Autodesk Fusion 360 part; units mm, degrees
(part 2 of 2)
sketch "Sketch13" plane through (0, 16, 0) normal (0, 1, 0) x (-1, 0, 0)
  arc A0 (-64.7977, -91.0875) -> (-65.2878, -90.2878) centre (-68, -92.5) ccw
  line L0 (-64.7977, -91.0875) -> (-65.3533, -91.0875)
  arc A1 (-65.3533, -91.0875) -> (-65.6435, -90.6435) centre (-68, -92.5) ccw
  line L1 (-65.6435, -90.6435) -> (-65.2878, -90.2878)
  arc A2 (-63.869, -96.131) -> (-62.7085, -94) centre (-68, -92.5) ccw
  line L2 (-63.869, -96.131) -> (-64.2233, -95.7767)
  arc A3 (-64.2233, -95.7767) -> (-63.2303, -94) centre (-68, -92.5) ccw
  line L3 (-63.2303, -94) -> (-62.7085, -94)
  arc A4 (-71.631, -96.631) -> (-64.369, -96.631) centre (-68, -92.5) ccw
  line L4 (-71.631, -96.631) -> (-71.2767, -96.2767)
  arc A5 (-71.2767, -96.2767) -> (-64.7233, -96.2767) centre (-68, -92.5) ccw
  line L5 (-64.7233, -96.2767) -> (-64.369, -96.631)
  line L6 (-69.9125, -91.0875) -> (-70.0627, -91.0875)
  arc A6 (-70, -91) -> (-70.0627, -91.0875) centre (-68, -92.5) ccw
  line L7 (-70, -91) -> (-69.9125, -91.0875)
  line L8 (-67.4952, -91.0875) -> (-68.5048, -91.0875)
  arc A7 (-67.4952, -91.0875) -> (-68.5048, -91.0875) centre (-68, -92.5) ccw
  arc A8 (-64.369, -88.369) -> (-71.631, -88.369) centre (-68, -92.5) ccw
  line L9 (-64.369, -88.369) -> (-64.7233, -88.7233)
  arc A9 (-64.7233, -88.7233) -> (-71.2767, -88.7233) centre (-68, -92.5) ccw
  line L10 (-71.2767, -88.7233) -> (-71.631, -88.369)
  arc A10 (-58.9221, -95.9221) -> (-53.0779, -95.9221) centre (-56, -92.5) ccw
  line L11 (-58.9221, -95.9221) -> (-58.5674, -95.5674)
  arc A11 (-58.5674, -95.5674) -> (-53.4326, -95.5674) centre (-56, -92.5) ccw
  line L12 (-53.4326, -95.5674) -> (-53.0779, -95.9221)
  arc A12 (-60.2426, -94) -> (-59.4221, -95.4221) centre (-56, -92.5) ccw
  line L13 (-60.2426, -94) -> (-59.7081, -94)
  arc A13 (-59.7081, -94) -> (-59.0674, -95.0674) centre (-56, -92.5) ccw
  line L14 (-59.0674, -95.0674) -> (-59.4221, -95.4221)
  line L15 (-43.4952, -91.0875) -> (-44.5048, -91.0875)
  arc A14 (-43.4952, -91.0875) -> (-44.5048, -91.0875) centre (-44, -92.5) ccw
  line L16 (-54.0875, -91.0875) -> (-54, -91)
  arc A15 (-53.9373, -91.0875) -> (-54, -91) centre (-56, -92.5) ccw
  line L17 (-53.9373, -91.0875) -> (-54.0875, -91.0875)
  arc A16 (-51.869, -96.131) -> (-50.7085, -94) centre (-56, -92.5) ccw
  line L18 (-51.869, -96.131) -> (-52.2233, -95.7767)
  arc A17 (-52.2233, -95.7767) -> (-51.2303, -94) centre (-56, -92.5) ccw
  line L19 (-51.2303, -94) -> (-50.7085, -94)
  arc A18 (-52.369, -88.369) -> (-59.631, -88.369) centre (-56, -92.5) ccw
  line L20 (-52.369, -88.369) -> (-52.7233, -88.7233)
  arc A19 (-52.7233, -88.7233) -> (-59.2767, -88.7233) centre (-56, -92.5) ccw
  line L21 (-59.2767, -88.7233) -> (-59.631, -88.369)
  line L22 (-41.9373, -91.0875) -> (-42.0875, -91.0875)
  line L23 (-42.0875, -91.0875) -> (-42, -91)
  arc A20 (-41.9373, -91.0875) -> (-42, -91) centre (-44, -92.5) ccw
  line L24 (-45.9125, -91.0875) -> (-46.0627, -91.0875)
  arc A21 (-46, -91) -> (-46.0627, -91.0875) centre (-44, -92.5) ccw
  line L25 (-46, -91) -> (-45.9125, -91.0875)
  arc A22 (-49.2915, -94) -> (-48.131, -96.131) centre (-44, -92.5) ccw
  line L26 (-49.2915, -94) -> (-48.7697, -94)
  arc A23 (-48.7697, -94) -> (-47.7767, -95.7767) centre (-44, -92.5) ccw
  line L27 (-47.7767, -95.7767) -> (-48.131, -96.131)
  arc A24 (-45.5, -94.5) -> (-42.5, -94.5) centre (-44, -92.5) ccw
  line L28 (-45.5, -94.5) -> (-45.1419, -94.1419)
  arc A25 (-45.1419, -94.1419) -> (-42.8581, -94.1419) centre (-44, -92.5) ccw
  line L29 (-42.8581, -94.1419) -> (-42.5, -94.5)
  arc A26 (-40.369, -88.369) -> (-47.631, -88.369) centre (-44, -92.5) ccw
  line L30 (-40.369, -88.369) -> (-40.7233, -88.7233)
  arc A27 (-40.7233, -88.7233) -> (-47.2767, -88.7233) centre (-44, -92.5) ccw
  line L31 (-47.2767, -88.7233) -> (-47.631, -88.369)
  arc A28 (-38.6845, -91.0875) -> (-39.869, -88.869) centre (-44, -92.5) ccw
  line L32 (-38.6845, -91.0875) -> (-39.2037, -91.0875)
  arc A29 (-39.2037, -91.0875) -> (-40.2233, -89.2233) centre (-44, -92.5) ccw
  line L33 (-40.2233, -89.2233) -> (-39.869, -88.869)
  arc A30 (-42.5, -90.5) -> (-45.5, -90.5) centre (-44, -92.5) ccw
  line L34 (-42.5, -90.5) -> (-42.8581, -90.8581)
  arc A31 (-42.8581, -90.8581) -> (-45.1419, -90.8581) centre (-44, -92.5) ccw
  line L35 (-45.1419, -90.8581) -> (-45.5, -90.5)
  arc A32 (-47.631, -96.631) -> (-40.369, -96.631) centre (-44, -92.5) ccw
  line L36 (-47.631, -96.631) -> (-47.2767, -96.2767)
  arc A33 (-47.2767, -96.2767) -> (-40.7233, -96.2767) centre (-44, -92.5) ccw
  line L37 (-40.7233, -96.2767) -> (-40.369, -96.631)
  arc A34 (-46.7122, -90.2878) -> (-47.2023, -91.0875) centre (-44, -92.5) ccw
  line L38 (-46.7122, -90.2878) -> (-46.3565, -90.6435)
  arc A35 (-46.3565, -90.6435) -> (-46.6467, -91.0875) centre (-44, -92.5) ccw
  line L39 (-46.6467, -91.0875) -> (-47.2023, -91.0875)
  arc A36 (-40.7977, -91.0875) -> (-41.2878, -90.2878) centre (-44, -92.5) ccw
  line L40 (-40.7977, -91.0875) -> (-41.3533, -91.0875)
  arc A37 (-41.3533, -91.0875) -> (-41.6435, -90.6435) centre (-44, -92.5) ccw
  line L41 (-41.6435, -90.6435) -> (-41.2878, -90.2878)
  arc A38 (-41.2878, -94.7122) -> (-40.8377, -94) centre (-44, -92.5) ccw
  line L42 (-41.2878, -94.7122) -> (-41.6435, -94.3565)
  arc A39 (-41.6435, -94.3565) -> (-41.4019, -94) centre (-44, -92.5) ccw
  line L43 (-41.4019, -94) -> (-40.8377, -94)
  arc A40 (-59.631, -96.631) -> (-52.369, -96.631) centre (-56, -92.5) ccw
  line L44 (-59.631, -96.631) -> (-59.2767, -96.2767)
  arc A41 (-59.2767, -96.2767) -> (-52.7233, -96.2767) centre (-56, -92.5) ccw
  line L45 (-52.7233, -96.2767) -> (-52.369, -96.631)
  arc A42 (-52.7977, -91.0875) -> (-53.2878, -90.2878) centre (-56, -92.5) ccw
  line L46 (-52.7977, -91.0875) -> (-53.3533, -91.0875)
  arc A43 (-53.3533, -91.0875) -> (-53.6435, -90.6435) centre (-56, -92.5) ccw
  line L47 (-53.6435, -90.6435) -> (-53.2878, -90.2878)
  arc A44 (-54.8581, -90.8581) -> (-57.1419, -90.8581) centre (-56, -92.5) ccw
  line L48 (-57.1419, -90.8581) -> (-57.5, -90.5)
  arc A45 (-54.5, -90.5) -> (-57.5, -90.5) centre (-56, -92.5) ccw
  line L49 (-54.5, -90.5) -> (-54.8581, -90.8581)
  line L50 (-57.9125, -91.0875) -> (-58.0627, -91.0875)
  arc A46 (-58, -91) -> (-58.0627, -91.0875) centre (-56, -92.5) ccw
  line L51 (-58, -91) -> (-57.9125, -91.0875)
  arc A47 (-58.2122, -95.2122) -> (-53.7878, -95.2122) centre (-56, -92.5) ccw
  line L52 (-58.2122, -95.2122) -> (-57.8565, -94.8565)
  arc A48 (-57.8565, -94.8565) -> (-54.1435, -94.8565) centre (-56, -92.5) ccw
  line L53 (-54.1435, -94.8565) -> (-53.7878, -95.2122)
  line L54 (-55.4952, -91.0875) -> (-56.5048, -91.0875)
  arc A49 (-55.4952, -91.0875) -> (-56.5048, -91.0875) centre (-56, -92.5) ccw
  arc A50 (-66.8581, -90.8581) -> (-69.1419, -90.8581) centre (-68, -92.5) ccw
  line L55 (-69.1419, -90.8581) -> (-69.5, -90.5)
  arc A51 (-66.5, -90.5) -> (-69.5, -90.5) centre (-68, -92.5) ccw
  line L56 (-66.5, -90.5) -> (-66.8581, -90.8581)
  arc A52 (-70.7122, -90.2878) -> (-71.2023, -91.0875) centre (-68, -92.5) ccw
  line L57 (-70.7122, -90.2878) -> (-70.3565, -90.6435)
  arc A53 (-70.3565, -90.6435) -> (-70.6467, -91.0875) centre (-68, -92.5) ccw
  line L58 (-70.6467, -91.0875) -> (-71.2023, -91.0875)
  arc A54 (-71.1623, -94) -> (-70.7122, -94.7122) centre (-68, -92.5) ccw
  line L59 (-71.1623, -94) -> (-70.5981, -94)
  arc A55 (-70.5981, -94) -> (-70.3565, -94.3565) centre (-68, -92.5) ccw
  line L60 (-70.3565, -94.3565) -> (-70.7122, -94.7122)
  arc A56 (-69.5, -94.5) -> (-66.5, -94.5) centre (-68, -92.5) ccw
  line L61 (-69.5, -94.5) -> (-69.1419, -94.1419)
  arc A57 (-69.1419, -94.1419) -> (-66.8581, -94.1419) centre (-68, -92.5) ccw
  line L62 (-66.8581, -94.1419) -> (-66.5, -94.5)
  line L63 (-66.0875, -91.0875) -> (-66, -91)
  arc A58 (-65.9373, -91.0875) -> (-66, -91) centre (-68, -92.5) ccw
  line L64 (-65.9373, -91.0875) -> (-66.0875, -91.0875)
  arc A59 (-63.7274, -91.0875) -> (-64.5779, -89.5779) centre (-68, -92.5) ccw
  line L65 (-63.7274, -91.0875) -> (-64.2577, -91.0875)
  arc A60 (-64.2577, -91.0875) -> (-64.9326, -89.9326) centre (-68, -92.5) ccw
  line L66 (-64.9326, -89.9326) -> (-64.5779, -89.5779)
  arc A61 (-64.5779, -95.4221) -> (-63.7574, -94) centre (-68, -92.5) ccw
  line L67 (-64.5779, -95.4221) -> (-64.9326, -95.0674)
  arc A62 (-64.9326, -95.0674) -> (-64.2919, -94) centre (-68, -92.5) ccw
  line L68 (-64.2919, -94) -> (-63.7574, -94)
  arc A63 (-70.9221, -95.9221) -> (-65.0779, -95.9221) centre (-68, -92.5) ccw
  line L69 (-70.9221, -95.9221) -> (-70.5674, -95.5674)
  arc A64 (-70.5674, -95.5674) -> (-65.4326, -95.5674) centre (-68, -92.5) ccw
  line L70 (-65.4326, -95.5674) -> (-65.0779, -95.9221)
  arc A65 (-73.2915, -94) -> (-72.131, -96.131) centre (-68, -92.5) ccw
  line L71 (-73.2915, -94) -> (-72.7697, -94)
  arc A66 (-72.7697, -94) -> (-71.7767, -95.7767) centre (-68, -92.5) ccw
  line L72 (-71.7767, -95.7767) -> (-72.131, -96.131)
  arc A67 (-72.131, -88.869) -> (-73.3155, -91.0875) centre (-68, -92.5) ccw
  line L73 (-72.131, -88.869) -> (-71.7767, -89.2233)
  arc A68 (-71.7767, -89.2233) -> (-72.7963, -91.0875) centre (-68, -92.5) ccw
  line L74 (-72.7963, -91.0875) -> (-73.3155, -91.0875)
  arc A69 (-65.4326, -89.4326) -> (-70.5674, -89.4326) centre (-68, -92.5) ccw
  line L75 (-70.5674, -89.4326) -> (-70.9221, -89.0779)
  arc A70 (-65.0779, -89.0779) -> (-70.9221, -89.0779) centre (-68, -92.5) ccw
  line L76 (-65.0779, -89.0779) -> (-65.4326, -89.4326)
  arc A71 (-52.5779, -95.4221) -> (-51.7574, -94) centre (-56, -92.5) ccw
  line L77 (-52.5779, -95.4221) -> (-52.9326, -95.0674)
  arc A72 (-52.9326, -95.0674) -> (-52.2919, -94) centre (-56, -92.5) ccw
  line L78 (-52.2919, -94) -> (-51.7574, -94)
  arc A73 (-59.1623, -94) -> (-58.7122, -94.7122) centre (-56, -92.5) ccw
  line L79 (-59.1623, -94) -> (-58.5981, -94)
  arc A74 (-58.5981, -94) -> (-58.3565, -94.3565) centre (-56, -92.5) ccw
  line L80 (-58.3565, -94.3565) -> (-58.7122, -94.7122)
  arc A75 (-59.4221, -89.5779) -> (-60.2726, -91.0875) centre (-56, -92.5) ccw
  line L81 (-59.4221, -89.5779) -> (-59.0674, -89.9326)
  arc A76 (-59.0674, -89.9326) -> (-59.7423, -91.0875) centre (-56, -92.5) ccw
  line L82 (-59.7423, -91.0875) -> (-60.2726, -91.0875)
  arc A77 (-53.4326, -89.4326) -> (-58.5674, -89.4326) centre (-56, -92.5) ccw
  line L83 (-58.5674, -89.4326) -> (-58.9221, -89.0779)
  arc A78 (-53.0779, -89.0779) -> (-58.9221, -89.0779) centre (-56, -92.5) ccw
  line L84 (-53.0779, -89.0779) -> (-53.4326, -89.4326)
  arc A79 (-50.6845, -91.0875) -> (-51.869, -88.869) centre (-56, -92.5) ccw
  line L85 (-50.6845, -91.0875) -> (-51.2037, -91.0875)
  arc A80 (-51.2037, -91.0875) -> (-52.2233, -89.2233) centre (-56, -92.5) ccw
  line L86 (-52.2233, -89.2233) -> (-51.869, -88.869)
  arc A81 (-60.131, -88.869) -> (-61.3155, -91.0875) centre (-56, -92.5) ccw
  line L87 (-60.131, -88.869) -> (-59.7767, -89.2233)
  arc A82 (-59.7767, -89.2233) -> (-60.7963, -91.0875) centre (-56, -92.5) ccw
  line L88 (-60.7963, -91.0875) -> (-61.3155, -91.0875)
  arc A83 (-39.7274, -91.0875) -> (-40.5779, -89.5779) centre (-44, -92.5) ccw
  line L89 (-39.7274, -91.0875) -> (-40.2577, -91.0875)
  arc A84 (-40.2577, -91.0875) -> (-40.9326, -89.9326) centre (-44, -92.5) ccw
  line L90 (-40.9326, -89.9326) -> (-40.5779, -89.5779)
  arc A85 (-47.1623, -94) -> (-46.7122, -94.7122) centre (-44, -92.5) ccw
  line L91 (-47.1623, -94) -> (-46.5981, -94)
  arc A86 (-46.5981, -94) -> (-46.3565, -94.3565) centre (-44, -92.5) ccw
  line L92 (-46.3565, -94.3565) -> (-46.7122, -94.7122)
  arc A87 (-48.131, -88.869) -> (-49.3155, -91.0875) centre (-44, -92.5) ccw
  line L93 (-48.131, -88.869) -> (-47.7767, -89.2233)
  arc A88 (-47.7767, -89.2233) -> (-48.7963, -91.0875) centre (-44, -92.5) ccw
  line L94 (-48.7963, -91.0875) -> (-49.3155, -91.0875)
  arc A89 (-46.2122, -95.2122) -> (-41.7878, -95.2122) centre (-44, -92.5) ccw
  line L95 (-46.2122, -95.2122) -> (-45.8565, -94.8565)
  arc A90 (-45.8565, -94.8565) -> (-42.1435, -94.8565) centre (-44, -92.5) ccw
  line L96 (-42.1435, -94.8565) -> (-41.7878, -95.2122)
  arc A91 (-41.0779, -89.0779) -> (-46.9221, -89.0779) centre (-44, -92.5) ccw
  line L97 (-41.0779, -89.0779) -> (-41.4326, -89.4326)
  arc A92 (-41.4326, -89.4326) -> (-46.5674, -89.4326) centre (-44, -92.5) ccw
  line L98 (-46.5674, -89.4326) -> (-46.9221, -89.0779)
  arc A93 (-39.869, -96.131) -> (-38.7085, -94) centre (-44, -92.5) ccw
  line L99 (-39.869, -96.131) -> (-40.2233, -95.7767)
  arc A94 (-40.2233, -95.7767) -> (-39.2303, -94) centre (-44, -92.5) ccw
  line L100 (-39.2303, -94) -> (-38.7085, -94)
  arc A95 (-41.7878, -89.7878) -> (-46.2122, -89.7878) centre (-44, -92.5) ccw
  line L101 (-41.7878, -89.7878) -> (-42.1435, -90.1435)
  arc A96 (-42.1435, -90.1435) -> (-45.8565, -90.1435) centre (-44, -92.5) ccw
  line L102 (-45.8565, -90.1435) -> (-46.2122, -89.7878)
  arc A97 (-46.9221, -95.9221) -> (-41.0779, -95.9221) centre (-44, -92.5) ccw
  line L103 (-46.9221, -95.9221) -> (-46.5674, -95.5674)
  arc A98 (-46.5674, -95.5674) -> (-41.4326, -95.5674) centre (-44, -92.5) ccw
  line L104 (-41.4326, -95.5674) -> (-41.0779, -95.9221)
  arc A99 (-47.4221, -89.5779) -> (-48.2726, -91.0875) centre (-44, -92.5) ccw
  line L105 (-47.4221, -89.5779) -> (-47.0674, -89.9326)
  arc A100 (-47.0674, -89.9326) -> (-47.7423, -91.0875) centre (-44, -92.5) ccw
  line L106 (-47.7423, -91.0875) -> (-48.2726, -91.0875)
  arc A101 (-48.2426, -94) -> (-47.4221, -95.4221) centre (-44, -92.5) ccw
  line L107 (-48.2426, -94) -> (-47.7081, -94)
  arc A102 (-47.7081, -94) -> (-47.0674, -95.0674) centre (-44, -92.5) ccw
  line L108 (-47.0674, -95.0674) -> (-47.4221, -95.4221)
  arc A103 (-40.5779, -95.4221) -> (-39.7574, -94) centre (-44, -92.5) ccw
  line L109 (-40.5779, -95.4221) -> (-40.9326, -95.0674)
  arc A104 (-40.9326, -95.0674) -> (-40.2919, -94) centre (-44, -92.5) ccw
  line L110 (-40.2919, -94) -> (-39.7574, -94)
  arc A105 (-61.2915, -94) -> (-60.131, -96.131) centre (-56, -92.5) ccw
  line L111 (-61.2915, -94) -> (-60.7697, -94)
  arc A106 (-60.7697, -94) -> (-59.7767, -95.7767) centre (-56, -92.5) ccw
  line L112 (-59.7767, -95.7767) -> (-60.131, -96.131)
  arc A107 (-51.7274, -91.0875) -> (-52.5779, -89.5779) centre (-56, -92.5) ccw
  line L113 (-51.7274, -91.0875) -> (-52.2577, -91.0875)
  arc A108 (-52.2577, -91.0875) -> (-52.9326, -89.9326) centre (-56, -92.5) ccw
  line L114 (-52.9326, -89.9326) -> (-52.5779, -89.5779)
  arc A109 (-54.1435, -90.1435) -> (-57.8565, -90.1435) centre (-56, -92.5) ccw
  line L115 (-57.8565, -90.1435) -> (-58.2122, -89.7878)
  arc A110 (-53.7878, -89.7878) -> (-58.2122, -89.7878) centre (-56, -92.5) ccw
  line L116 (-53.7878, -89.7878) -> (-54.1435, -90.1435)
  arc A111 (-58.7122, -90.2878) -> (-59.2023, -91.0875) centre (-56, -92.5) ccw
  line L117 (-58.7122, -90.2878) -> (-58.3565, -90.6435)
  arc A112 (-58.3565, -90.6435) -> (-58.6467, -91.0875) centre (-56, -92.5) ccw
  line L118 (-58.6467, -91.0875) -> (-59.2023, -91.0875)
  arc A113 (-57.5, -94.5) -> (-54.5, -94.5) centre (-56, -92.5) ccw
  line L119 (-57.5, -94.5) -> (-57.1419, -94.1419)
  arc A114 (-57.1419, -94.1419) -> (-54.8581, -94.1419) centre (-56, -92.5) ccw
  line L120 (-54.8581, -94.1419) -> (-54.5, -94.5)
  arc A115 (-53.2878, -94.7122) -> (-52.8377, -94) centre (-56, -92.5) ccw
  line L121 (-53.2878, -94.7122) -> (-53.6435, -94.3565)
  arc A116 (-53.6435, -94.3565) -> (-53.4019, -94) centre (-56, -92.5) ccw
  line L122 (-53.4019, -94) -> (-52.8377, -94)
  arc A117 (-66.1435, -90.1435) -> (-69.8565, -90.1435) centre (-68, -92.5) ccw
  line L123 (-69.8565, -90.1435) -> (-70.2122, -89.7878)
  arc A118 (-65.7878, -89.7878) -> (-70.2122, -89.7878) centre (-68, -92.5) ccw
  line L124 (-65.7878, -89.7878) -> (-66.1435, -90.1435)
  arc A119 (-71.4221, -89.5779) -> (-72.2726, -91.0875) centre (-68, -92.5) ccw
  line L125 (-71.4221, -89.5779) -> (-71.0674, -89.9326)
  arc A120 (-71.0674, -89.9326) -> (-71.7423, -91.0875) centre (-68, -92.5) ccw
  line L126 (-71.7423, -91.0875) -> (-72.2726, -91.0875)
  arc A121 (-72.2426, -94) -> (-71.4221, -95.4221) centre (-68, -92.5) ccw
  line L127 (-72.2426, -94) -> (-71.7081, -94)
  arc A122 (-71.7081, -94) -> (-71.0674, -95.0674) centre (-68, -92.5) ccw
  line L128 (-71.0674, -95.0674) -> (-71.4221, -95.4221)
  arc A123 (-70.2122, -95.2122) -> (-65.7878, -95.2122) centre (-68, -92.5) ccw
  line L129 (-70.2122, -95.2122) -> (-69.8565, -94.8565)
  arc A124 (-69.8565, -94.8565) -> (-66.1435, -94.8565) centre (-68, -92.5) ccw
  line L130 (-66.1435, -94.8565) -> (-65.7878, -95.2122)
  arc A125 (-65.2878, -94.7122) -> (-64.8377, -94) centre (-68, -92.5) ccw
  line L131 (-65.2878, -94.7122) -> (-65.6435, -94.3565)
  arc A126 (-65.6435, -94.3565) -> (-65.4019, -94) centre (-68, -92.5) ccw
  line L132 (-65.4019, -94) -> (-64.8377, -94)
  arc A127 (-62.6845, -91.0875) -> (-63.869, -88.869) centre (-68, -92.5) ccw
  line L133 (-62.6845, -91.0875) -> (-63.2037, -91.0875)
  arc A128 (-63.2037, -91.0875) -> (-64.2233, -89.2233) centre (-68, -92.5) ccw
  line L134 (-64.2233, -89.2233) -> (-63.869, -88.869)
  line L135 (-75, 0) -> (-70, 0)
  line L136 (-70, 0) -> (-65, -5)
  line L137 (-65, -5) -> (-70, -5)
  line L138 (-70, -5) -> (-75, 0)
  line L139 (-35, 0) -> (-30, 0)
  line L140 (-30, 0) -> (-25, -5)
  line L141 (-25, -5) -> (-30, -5)
  line L142 (-30, -5) -> (-35, 0)
  line L143 (-5, 0) -> (0, 0)
  line L144 (0, 0) -> (0, -5)
  line L145 (0, -5) -> (-5, 0)
  line L146 (-45, 0) -> (-40, 0)
  line L147 (-40, 0) -> (-35, -5)
  line L148 (-35, -5) -> (-40, -5)
  line L149 (-40, -5) -> (-45, 0)
  line L150 (-85, 0) -> (-80, 0)
  line L151 (-80, 0) -> (-75, -5)
  line L152 (-75, -5) -> (-80, -5)
  line L153 (-80, -5) -> (-85, 0)
  line L154 (-65, 0) -> (-60, 0)
  line L155 (-60, 0) -> (-55, -5)
  line L156 (-55, -5) -> (-60, -5)
  line L157 (-60, -5) -> (-65, 0)
  line L158 (-25, 0) -> (-20, 0)
  line L159 (-20, 0) -> (-15, -5)
  line L160 (-15, -5) -> (-20, -5)
  line L161 (-20, -5) -> (-25, 0)
  line L162 (-15, 0) -> (-10, 0)
  line L163 (-10, 0) -> (-5, -5)
  line L164 (-5, -5) -> (-10, -5)
  line L165 (-10, -5) -> (-15, 0)
  line L166 (-55, 0) -> (-50, 0)
  line L167 (-50, 0) -> (-45, -5)
  line L168 (-45, -5) -> (-50, -5)
  line L169 (-50, -5) -> (-55, 0)
  line L170 (-90, 0) -> (-85.1002, -5)
  line L171 (-85.1002, -5) -> (-90, -5)
  line L172 (-90, -5) -> (-90, 0)
  line L173 (-89, -87) -> (-87, -85.23)
  line L174 (-87, -85.23) -> (-85, -85.23)
  line L175 (-85, -85.23) -> (-85, -83)
  line L176 (-85, -83) -> (-83, -81)
  line L177 (-83, -81) -> (-83, -87)
  line L178 (-83, -87) -> (-89, -87)
  line L179 (-98, -90) -> (-100, -91.8748)
  line L180 (-100, -91.8748) -> (-100, -70)
  line L181 (-100, -70) -> (-78.1115, -70)
  line L182 (-78.1115, -70) -> (-80, -72)
  line L183 (-80, -72) -> (-98, -72)
  line L184 (-98, -72) -> (-98, -90)
  line L185 (-81, -89) -> (-81, -79)
  line L186 (-81, -79) -> (-79, -77)
  line L187 (-79, -77) -> (-79, -91)
  line L188 (-79, -91) -> (-93, -91)
  line L189 (-93, -91) -> (-91, -89)
  line L190 (-91, -89) -> (-81, -89)
  line L191 (-92, -84) -> (-92, -78)
  line L192 (-92, -78) -> (-86, -78)
  line L193 (-86, -78) -> (-88, -80)
  line L194 (-88, -80) -> (-90.23, -80)
  line L195 (-90.23, -80) -> (-90.23, -82)
  line L196 (-90.23, -82) -> (-92, -84)
  line L197 (-94, -86) -> (-96, -88)
  line L198 (-96, -88) -> (-96, -74)
  line L199 (-96, -74) -> (-82, -74)
  line L200 (-82, -74) -> (-84, -76)
  line L201 (-84, -76) -> (-94, -76)
  line L202 (-94, -76) -> (-94, -86)
  line L203 (-77, -93) -> (-77, -75)
  line L204 (-77, -75) -> (-75, -73.1115)
  line L205 (-75, -73.1115) -> (-75, -95)
  line L206 (-75, -95) -> (-96.8748, -95)
  line L207 (-96.8748, -95) -> (-95, -93)
  line L208 (-95, -93) -> (-77, -93)
  arc A129 (-103.4, 10) -> (-108.4, 5) centre (-103.4, 5) ccw
  line L209 (-108.4, 5) -> (-108.4, -104.18)
  arc A130 (-108.4, -104.18) -> (-103.4, -109.18) centre (-103.4, -104.18) ccw
  line L210 (-103.4, -109.18) -> (5, -109.18)
  arc A131 (5, -109.18) -> (10, -104.18) centre (5, -104.18) ccw
  line L211 (10, -104.18) -> (10, 5)
  arc A132 (10, 5) -> (5, 10) centre (5, 5) ccw
  line L212 (5, 10) -> (-103.4, 10)
  line L213 (-0.6538, -15.4306) -> (-0.6538, -90.1906)
  arc A133 (-5.6538, -95.1906) -> (-0.6538, -90.1906) centre (-5.6538, -90.1906) ccw
  line L214 (-5.6538, -95.1906) -> (-31.0838, -95.1906)
  arc A134 (-36.0838, -90.1906) -> (-31.0838, -95.1906) centre (-31.0838, -90.1906) ccw
  line L215 (-36.0838, -90.1906) -> (-36.0838, -15.4306)
  arc A135 (-31.0838, -10.4306) -> (-36.0838, -15.4306) centre (-31.0838, -15.4306) ccw
  line L216 (-31.0838, -10.4306) -> (-5.6538, -10.4306)
  arc A136 (-0.6538, -15.4306) -> (-5.6538, -10.4306) centre (-5.6538, -15.4306) ccw
  line L217 (-65.22, -73.425) -> (-39.72, -73.425)
  arc A137 (-37.72, -75.425) -> (-39.72, -73.425) centre (-39.72, -75.425) ccw
  line L218 (-37.72, -75.425) -> (-37.72, -83.425)
  arc A138 (-39.72, -85.425) -> (-37.72, -83.425) centre (-39.72, -83.425) ccw
  line L219 (-39.72, -85.425) -> (-65.22, -85.425)
  arc A139 (-67.22, -83.425) -> (-65.22, -85.425) centre (-65.22, -83.425) ccw
  line L220 (-67.22, -83.425) -> (-67.22, -75.425)
  arc A140 (-65.22, -73.425) -> (-67.22, -75.425) centre (-65.22, -75.425) ccw
  circle A141 centre (-103.4, -104.18) radius 1.45
  circle A142 centre (-103.4, 5) radius 1.45
  circle A143 centre (5, -104.18) radius 1.45
  circle A144 centre (5, 5) radius 1.45
  line L221 (-93.99, -14.314) -> (-80.99, -14.314)
  line L222 (-93.99, -28.314) -> (-80.99, -28.314)
  line L223 (-94.49, -14.814) -> (-94.49, -27.814)
  line L224 (-80.49, -14.814) -> (-80.49, -27.814)
  arc A145 (-93.99, -14.314) -> (-94.49, -14.814) centre (-93.99, -14.814) ccw
  arc A146 (-80.49, -14.814) -> (-80.99, -14.314) centre (-80.99, -14.814) ccw
  arc A147 (-94.49, -27.814) -> (-93.99, -28.314) centre (-93.99, -27.814) ccw
  arc A148 (-80.99, -28.314) -> (-80.49, -27.814) centre (-80.99, -27.814) ccw
  line L225 (-74.94, -14.314) -> (-61.94, -14.314)
  line L226 (-74.94, -28.314) -> (-61.94, -28.314)
  line L227 (-75.44, -14.814) -> (-75.44, -27.814)
  line L228 (-61.44, -14.814) -> (-61.44, -27.814)
  arc A149 (-74.94, -14.314) -> (-75.44, -14.814) centre (-74.94, -14.814) ccw
  arc A150 (-61.44, -14.814) -> (-61.94, -14.314) centre (-61.94, -14.814) ccw
  arc A151 (-75.44, -27.814) -> (-74.94, -28.314) centre (-74.94, -27.814) ccw
  arc A152 (-61.94, -28.314) -> (-61.44, -27.814) centre (-61.94, -27.814) ccw
  line L229 (-55.89, -14.314) -> (-42.89, -14.314)
  line L230 (-55.89, -28.314) -> (-42.89, -28.314)
  line L231 (-56.39, -14.814) -> (-56.39, -27.814)
  line L232 (-42.39, -14.814) -> (-42.39, -27.814)
  arc A153 (-55.89, -14.314) -> (-56.39, -14.814) centre (-55.89, -14.814) ccw
  arc A154 (-42.39, -14.814) -> (-42.89, -14.314) centre (-42.89, -14.814) ccw
  arc A155 (-56.39, -27.814) -> (-55.89, -28.314) centre (-55.89, -27.814) ccw
  arc A156 (-42.89, -28.314) -> (-42.39, -27.814) centre (-42.89, -27.814) ccw
  line L233 (-93.99, -33.364) -> (-80.99, -33.364)
  line L234 (-93.99, -47.364) -> (-80.99, -47.364)
  line L235 (-94.49, -33.864) -> (-94.49, -46.864)
  line L236 (-80.49, -33.864) -> (-80.49, -46.864)
  arc A157 (-93.99, -33.364) -> (-94.49, -33.864) centre (-93.99, -33.864) ccw
  arc A158 (-80.49, -33.864) -> (-80.99, -33.364) centre (-80.99, -33.864) ccw
  arc A159 (-94.49, -46.864) -> (-93.99, -47.364) centre (-93.99, -46.864) ccw
  arc A160 (-80.99, -47.364) -> (-80.49, -46.864) centre (-80.99, -46.864) ccw
  line L237 (-74.94, -33.364) -> (-61.94, -33.364)
  line L238 (-74.94, -47.364) -> (-61.94, -47.364)
  line L239 (-75.44, -33.864) -> (-75.44, -46.864)
  line L240 (-61.44, -33.864) -> (-61.44, -46.864)
  arc A161 (-74.94, -33.364) -> (-75.44, -33.864) centre (-74.94, -33.864) ccw
  arc A162 (-61.44, -33.864) -> (-61.94, -33.364) centre (-61.94, -33.864) ccw
  arc A163 (-75.44, -46.864) -> (-74.94, -47.364) centre (-74.94, -46.864) ccw
  arc A164 (-61.94, -47.364) -> (-61.44, -46.864) centre (-61.94, -46.864) ccw
  line L241 (-55.89, -33.364) -> (-42.89, -33.364)
  line L242 (-55.89, -47.364) -> (-42.89, -47.364)
  line L243 (-56.39, -33.864) -> (-56.39, -46.864)
  line L244 (-42.39, -33.864) -> (-42.39, -46.864)
  arc A165 (-55.89, -33.364) -> (-56.39, -33.864) centre (-55.89, -33.864) ccw
  arc A166 (-42.39, -33.864) -> (-42.89, -33.364) centre (-42.89, -33.864) ccw
  arc A167 (-56.39, -46.864) -> (-55.89, -47.364) centre (-55.89, -46.864) ccw
  arc A168 (-42.89, -47.364) -> (-42.39, -46.864) centre (-42.89, -46.864) ccw
  line L245 (-93.99, -52.414) -> (-80.99, -52.414)
  line L246 (-93.99, -66.414) -> (-80.99, -66.414)
  line L247 (-94.49, -52.914) -> (-94.49, -65.914)
  line L248 (-80.49, -52.914) -> (-80.49, -65.914)
  arc A169 (-93.99, -52.414) -> (-94.49, -52.914) centre (-93.99, -52.914) ccw
  arc A170 (-80.49, -52.914) -> (-80.99, -52.414) centre (-80.99, -52.914) ccw
  arc A171 (-94.49, -65.914) -> (-93.99, -66.414) centre (-93.99, -65.914) ccw
  arc A172 (-80.99, -66.414) -> (-80.49, -65.914) centre (-80.99, -65.914) ccw
  line L249 (-74.94, -52.414) -> (-61.94, -52.414)
  line L250 (-74.94, -66.414) -> (-61.94, -66.414)
  line L251 (-75.44, -52.914) -> (-75.44, -65.914)
  line L252 (-61.44, -52.914) -> (-61.44, -65.914)
  arc A173 (-74.94, -52.414) -> (-75.44, -52.914) centre (-74.94, -52.914) ccw
  arc A174 (-61.44, -52.914) -> (-61.94, -52.414) centre (-61.94, -52.914) ccw
  arc A175 (-75.44, -65.914) -> (-74.94, -66.414) centre (-74.94, -65.914) ccw
  arc A176 (-61.94, -66.414) -> (-61.44, -65.914) centre (-61.94, -65.914) ccw
  line L253 (-55.89, -52.414) -> (-42.89, -52.414)
  line L254 (-55.89, -66.414) -> (-42.89, -66.414)
  line L255 (-56.39, -52.914) -> (-56.39, -65.914)
  line L256 (-42.39, -52.914) -> (-42.39, -65.914)
  arc A177 (-55.89, -52.414) -> (-56.39, -52.914) centre (-55.89, -52.914) ccw
  arc A178 (-42.39, -52.914) -> (-42.89, -52.414) centre (-42.89, -52.914) ccw
  arc A179 (-56.39, -65.914) -> (-55.89, -66.414) centre (-55.89, -65.914) ccw
  arc A180 (-42.89, -66.414) -> (-42.39, -65.914) centre (-42.89, -65.914) ccw
  line L257 (-97.015, -68.939) -> (-39.865, -68.939)
  line L258 (-97.015, -11.789) -> (-39.865, -11.789)
  line L259 (-97.015, -68.939) -> (-97.015, -11.789)
  line L260 (-39.865, -68.939) -> (-39.865, -11.789)
extrude "Extrude13" cut sketch "Sketch13" against normal blind 3 contours L221 L222 L223 L224 A145 A146 A147 A148 | L225 L226 L227 L228 A149 A150 A151 A152 | L229 L230 L231 L232 A153 A154 A155 A156 | L233 L234 L235 L236 A157 A158 A159 A160 | L237 L238 L239 L240 A161 A162 A163 A164 | L241 L242 L243 L244 A165 A166 A167 A168 | L245 L246 L247 L248 A169 A170 A171 A172 | L249 L250 L251 L252 A173 A174 A175 A176 | L253 L254 L255 L256 A177 A178 A179 A180 bodies 2
hidden bodies 1 3
